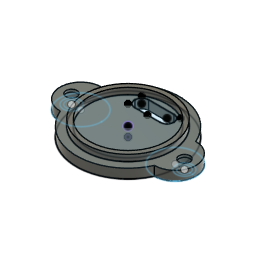
85c1-back-cover-type-c (Autodesk Fusion 360 design; units mm, degrees)
Autodesk Fusion 360 part; units mm, degrees
sketch "스케치1" plane through (0, 0, 0) normal (0, 1, 0) x (1, 0, 0)
  circle A0 centre (0, 0) radius 12.15
  circle A1 centre (11.15, 0) radius 4.9
  circle A2 centre (-11.15, 0) radius 4.9
  circle A3 centre (13.35, 0) radius 1.3
  circle A4 centre (-13.35, 0) radius 1.3
  circle A5 centre (13.35, 0) radius 1.925
  circle A6 centre (-13.35, 0) radius 1.925
  dimension "d1" = 24.3
  dimension "d2" = 9.8
  dimension "d3" = 9.8
  dimension "d4" = 2.6
  dimension "d5" = 2.2
  dimension "d6" = 2.6
  dimension "d7" = 2.2
  dimension "d8" = 11.15
  dimension "d9" = 11.15
  dimension "d10" = 3.85
  dimension "d11" = 3.85
  constraint coincident A0.centre origin
  constraint concentric A3 A5
  constraint concentric A4 A6
  measures "d1" diameter of A0
  measures "d2" diameter of A1
  measures "d3" diameter of A2
  measures "d4" diameter of A3
  measures "d5" distance of A1.centre A3.centre
  measures "d6" diameter of A4
  measures "d7" distance of A2.centre A4.centre
  measures "d8" distance of A0.centre A1.centre
  measures "d9" distance of A0.centre A2.centre
  measures "d10" diameter of A5
  measures "d11" diameter of A6
extrude "돌출1" add sketch "스케치1" along normal blind 2.2
extrude "돌출2" cut sketch "스케치1" along normal blind 1.6 contours A0 A4 A6 | A0 A4 A6 | A0 A4 | A0 A4
extrude "돌출3" cut sketch "스케치1" along normal blind 1.6 contours A0 A3 | A0 A3 A5 | A0 A3 A5 picked at (12.0867, 0.0541)
extrude "돌출4" cut sketch "스케치1" along normal blind 2.2 contours A0 A3 | A0 A3
extrude "돌출5" cut sketch "스케치1" along normal blind 2.2 contours A0 A4 | A0 A4
sketch "스케치2" plane through (0, 2.2, 0) normal (0, 1, 0) x (-1, 0, 0)
  circle A0 centre (13.35, 0) radius 1.3
  circle A1 centre (-13.35, 0) radius 1.3
  arc A2 (-11.1182, -4.8999) -> (11.1182, -4.8999) centre (0, 0) ccw
  arc A3 (11.1182, -4.8999) -> (11.1182, 4.8999) centre (11.15, 0) ccw
  arc A4 (11.1182, 4.8999) -> (-11.1182, 4.8999) centre (0, 0) ccw
  arc A5 (-11.1182, 4.8999) -> (-11.1182, -4.8999) centre (-11.15, 0) ccw
  circle A6 centre (0, 0) radius 10.25
  circle A7 centre (0, 0) radius 9.15
  dimension "d22" = 20.5
  dimension "d23" = 18.3
  constraint concentric A2 A6
  constraint concentric A6 A7
  measures "d22" diameter of A6
  measures "d23" diameter of A7
extrude "돌출6" add sketch "스케치2" along normal blind 1.5 contours A6
sketch "스케치3" plane through (0, 2.2, 0) normal (0, 1, 0) x (-1, 0, 0)
  circle A0 centre (0, 0) radius 9.15
  line L0 (3, -7.86) -> (-3, -7.86)
  line L1 (-4.6, -6.26) -> (-4.6, -6.2)
  line L2 (-3, -4.6) -> (3, -4.6)
  line L3 (4.6, -6.2) -> (4.6, -6.26)
  arc A1 (-4.6, -6.26) -> (-3, -7.86) centre (-3, -6.26) ccw
  arc A2 (-3, -4.6) -> (-4.6, -6.2) centre (-3, -6.2) ccw
  arc A3 (3, -7.86) -> (4.6, -6.26) centre (3, -6.26) ccw
  arc A4 (4.6, -6.2) -> (3, -4.6) centre (3, -6.2) ccw
  point P0 (4.6, -7.86)
  point P1 (-4.6, -7.86)
  point P2 (4.6, -4.6)
  point P3 (0, -4.6)
  dimension "d26" = 9.2
  dimension "d27" = 3.26
  dimension "d28" = 1.6
  dimension "d29" = 1.6
  dimension "d30" = 1.6
  dimension "d31" = 1.6
  dimension "d32" = 4.6
  constraint horizontal L0
  constraint vertical L1
  constraint horizontal L2
  constraint vertical L3
  constraint coincident P1 L0
  constraint coincident P1 L1
  constraint tangent L0 A1
  constraint tangent L1 A1
  constraint tangent L1 A2
  constraint tangent L2 A2
  constraint coincident P0 L0
  constraint coincident P0 L3
  constraint tangent L0 A3
  constraint tangent L3 A3
  constraint coincident P2 L2
  constraint coincident P2 L3
  constraint tangent L2 A4
  constraint tangent L3 A4
  constraint coincident L2 P3
  constraint midpoint L2 P3
  constraint vertical P3 A0.centre
  measures "d26" distance of P0 P1
  measures "d27" distance of P0 P2
  measures "d28" radius of A1
  measures "d29" radius of A2
  measures "d30" radius of A3
  measures "d31" radius of A4
  measures "d32" distance of A0.centre L2
extrude "돌출7" cut sketch "스케치3" against normal blind 10 contours L0 L1 L2 L3 A1 A2 A3 A4
